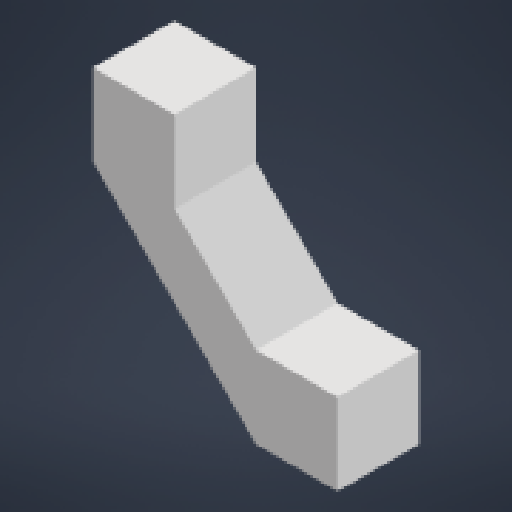
# Autodesk Inventor part: TriangleConnector
Saved by Autodesk Inventor 2027 (Build 310192000, 192)
## iProperties
Created: 2026-03-26
Part Number: TriangleConnector
Material: Generic
Document SubType Name: Modeling
Designer: Tueha
Density: 1 g/cm^3
Appearance: Default
Author: Tueha
Autodesk Inventor part; units mm, degrees
ref_plane "YZ Plane" through (0, 0, 0) normal (1, 0, 0) x (0, 1, 0)
ref_plane "XZ Plane" through (0, 0, 0) normal (0, 1, 0) x (-1, 0, 0)
ref_plane "XY Plane" through (0, 0, 0) normal (0, 0, 1) x (1, 0, 0)
sketch "Sketch1" plane through (0, 0, 0) normal (0, 0, 1) x (1, 0, 0)
  line L0 (-0.0466, 4.8213) -> (-6.0466, 4.8213)
  line L1 (-6.0466, 4.8213) -> (-6.0466, 10.8213)
  line L2 (-6.0466, 10.8213) -> (-0.0466, 10.8213)
  line L3 (-0.0466, 10.8213) -> (-0.0466, 4.8213)
  line L4 (-12.0466, 16.8213) -> (-18.0466, 16.8213)
  line L5 (-18.0466, 16.8213) -> (-18.0466, 22.8213)
  line L6 (-18.0466, 22.8213) -> (-12.0466, 22.8213)
  line L7 (-12.0466, 22.8213) -> (-12.0466, 16.8213)
  line L8 (-6.0466, 10.8213) -> (-12.0466, 16.8213)
  line L9 (-6.0466, 4.8213) -> (-18.0466, 16.8213)
  point P0 (0, 0)
  dimension "d0" = 6
  dimension "d1" = 6
  dimension "d4" = 6
  dimension "d5" = 6
  dimension "d6" = 45
  dimension "d7" = 6
  constraints: 20 end point, 4 parallel, 2 horizontal, 2 perpendicular
  measures "d0" distance of L2.end L0.start
  measures "d1" distance of L0.start L0.end
  measures "d4" distance of L6.end L4.start
  measures "d5" distance of L4.start L4.end
  measures "d6" angle of L9 L1
  measures "d7" distance between parallel lines of L2 L4
extrude "Extrusion1" add sketch "Sketch1" along normal blind 6
body "Solid1"
